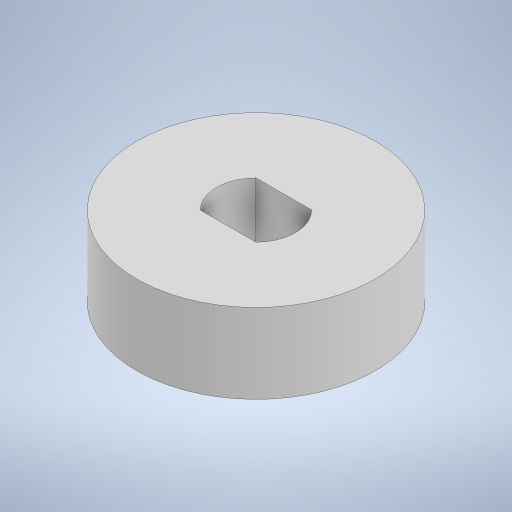
# Autodesk Inventor part: generic-launcher-blank
Saved by Autodesk Inventor 2023 (Build 270158030, 158C)
## iProperties
Created: 2024-09-20
Part Number: generic-launcher-blank
Material: Generic
Document SubType Name: Modeling
Designer: Imogen Heard
Density: 1 g/cm^3
Appearance: Default
Author: Imogen Heard
Autodesk Inventor part; units mm, degrees
ref_plane "YZ Plane" through (0, 0, 0) normal (1, 0, 0) x (0, 1, 0)
ref_plane "XZ Plane" through (0, 0, 0) normal (0, 1, 0) x (-1, 0, 0)
ref_plane "XY Plane" through (0, 0, 0) normal (0, 0, 1) x (1, 0, 0)
sketch "Sketch1" plane through (0, 0, 0) normal (0, 1, 0) x (-1, 0, 0)
  circle A0 centre (0, 0) radius 15
  dimension "d0" = 30
  constraints: 1 centre point, 1 coincident
  measures "d0" diameter of A0
extrude "Extrusion1" add sketch "Sketch1" along normal blind 10
sketch "Sketch2" plane through (0, 0, 0) normal (0, -1, 0) x (1, 0, 0)
  line L0 (-3.5, 3.5) -> (3.5, 3.5)
  line L1 (3.5, 3.5) -> (3.5, -3.5)
  line L2 (3.5, -3.5) -> (-3.5, -3.5)
  line L3 (-3.5, -3.5) -> (-3.5, 3.5)
  circle A0 centre (0, 0) radius 4.9497
  dimension "d3" = 7
  dimension "d4" = 7
  dimension "d5" = 3.5
  dimension "d6" = 3.5
  constraints: 8 end point, 2 parallel, 1 coincident, 1 horizontal, 1 perpendicular, 3 other
  measures "d3" distance between parallel lines of L2 L0
  measures "d4" distance between parallel lines of L3 L1
  measures "d5" distance from line of point (0, 0) L1
  measures "d6" distance from line of L2 point (0, 0)
extrude "Extrusion2" cut sketch "Sketch2" against normal blind 12.7 contours L0 L1 L2 L3 | L3 A0 | A0 L1
equation "\"d5\" = 0.5 * d4"
equation "\"d6\" = 0.5 * d3"
body "Solid1"
